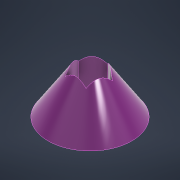
# Autodesk Inventor part: 1
Saved by Autodesk Inventor 2021.2 (Build 252289000, 289)
## iProperties
Created: 2023-09-06
Part Number: 1
Material: Типовые
Document SubType Name: Modeling
Designer: User
Density: 1 g/cm^3
Appearance: По умолчанию
Author: User
Autodesk Inventor part; units mm, degrees
ref_plane "YZ Plane" through (0, 0, 0) normal (1, 0, 0) x (0, 1, 0)
ref_plane "XZ Plane" through (0, 0, 0) normal (0, 1, 0) x (-1, 0, 0)
ref_plane "XY Plane" through (0, 0, 0) normal (0, 0, 1) x (1, 0, 0)
sketch "Эскиз1" plane through (0, 0, 0) normal (0, 0, 1) x (1, 0, 0)
  line L0 (0, 0) -> (10, 0)
  line L1 (10, 0) -> (0, 15.3986)
  line L2 (0, 15.3986) -> (0, 0)
  dimension "d0" = 10
  dimension "d1" = 57
  constraints: 6 end point, 1 horizontal, 1 perpendicular
  measures "d0" distance of L0.start L0.end
  measures "d1" angle of L1 L0
revolve "Вращение1" add sketch "Эскиз1" angle 360 about axis through (0, 15.3986, 0) along (0, -1, 0)
sketch "Эскиз2" plane through (0, 0, 0) normal (0, 1, 0) x (-1, 0, 0)
  line L0 (0, -4.2533) -> (-4.0451, -1.3143)
  line L1 (-4.0451, -1.3143) -> (-2.5, 3.441)
  line L2 (-2.5, 3.441) -> (2.5, 3.441)
  line L3 (2.5, 3.441) -> (4.0451, -1.3143)
  line L4 (4.0451, -1.3143) -> (0, -4.2533)
  point P0 (0, 0)
  point P1 (0, 0)
  dimension "d3" = 5
  constraints: 10 end point, 1 coincident, 11 other
  measures "d3" distance of L1.end L2.end
extrude "Выдавливание1" cut sketch "Эскиз2" along normal blind 40
